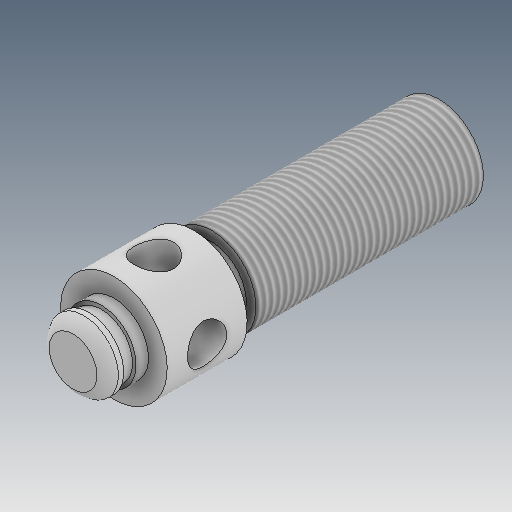
# Autodesk Inventor part: 螺杆
Saved by Autodesk Inventor 2020 (Build 240168000, 168)
## iProperties
Created: 2021-05-02
Part Number: 螺杆
Material: 常规
Document SubType Name: Modeling
Designer: Luorily
Density: 1 g/cm^3
Appearance: 默认
Author: Luorily
Autodesk Inventor part; units mm, degrees
ref_plane "YZ Plane" through (0, 0, 0) normal (1, 0, 0) x (0, 1, 0)
ref_plane "XZ Plane" through (0, 0, 0) normal (0, 1, 0) x (-1, 0, 0)
ref_plane "XY Plane" through (0, 0, 0) normal (0, 0, 1) x (1, 0, 0)
sketch "草图1" plane through (0, 0, 0) normal (1, 0, 0) x (0, 1, 0)
  line L0 (19.5, -23) -> (30, -23)
  line L1 (30, -23) -> (30, -68)
  line L2 (30, -68) -> (19.5, -68)
  line L3 (19.5, -68) -> (19.5, -78)
  line L4 (19.5, -78) -> (25, -78)
  line L5 (25, -78) -> (25, -206)
  line L6 (25, -206) -> (0, -206)
  line L7 (0, -206) -> (0, 0)
  line L8 (17.5, -16) -> (17.5, -9)
  line L9 (17.5, -9) -> (19.5, -9)
  line L10 (17.5, -16) -> (19.5, -16)
  line L11 (19.5, -16) -> (19.5, -23)
  line L12 (19.5, -23) -> (19.5, -6)
  line L13 (0, 0) -> (13.5, 0)
  arc A0 (19.5, -6) -> (13.5, 0) centre (8.1859, -11.3141) ccw
  dimension "d2" = 10.5
  dimension "d3" = 45
  dimension "d4" = 10.5
  dimension "d5" = 10
  dimension "d6" = 5.5
  dimension "d7" = 128
  dimension "d10" = 7
  dimension "d11" = 17
  dimension "d14" = 13.5
  dimension "d15" = 25
  constraints: 28 end point, 7 perpendicular, 2 parallel, 2 point on circle, 1 centre point, 1 horizontal
  measures "d2" distance of L0.start L0.end
  measures "d3" distance of L0.end L1.end
  measures "d4" distance of L1.end L2.end
  measures "d5" distance of L2.end L3.end
  measures "d6" distance of L3.end L4.end
  measures "d7" distance of L4.end L5.end
  measures "d10" distance of L8.start L8.end
  measures "d11" distance of L12.end L0.start
  measures "d14" distance of L7.end L13.end
  measures "d15" distance of L5.end L6.end
revolve "旋转1" add sketch "草图1" angle 360 about axis through (0, 0, -206) along (0, 0, 1) contours L0 L1 L2 L3 L4 L5 L6 L7 L13 A0 L12 L9 L8 L10 L11
sketch "草图2" plane through (0, 0, 0) normal (0, 1, 0) x (-1, 0, 0)
  line L0 (-19.5, -68) -> (19.5, -68) projected
  line L1 (0, -68) -> (0, -45.5)
  circle A0 centre (0, -45.5) radius 11
  point P0 (0, 0)
  dimension "d17" = 22.5
  dimension "d18" = 22
  constraints: 2 end point, 1 centre point, 1 coincident, 1 midpoint, 1 vertical
  measures "d17" distance of L1.start L1.end
  measures "d18" diameter of A0
extrude "拉伸1" cut sketch "草图2" along normal blind 100 and the other way blind 100
thread "螺纹1" size "M50x4" class "6g" standard "ANSI Metric M Profile" full length
sketch "草图3" plane through (0, 0, 0) normal (1, 0, 0) x (0, 1, 0)
  line L0 (-19.5, -68) -> (19.5, -68) projected
  line L1 (0, -68) -> (0, -45.5)
  circle A0 centre (0, -45.5) radius 11
  line L2 (-30, -34.5) -> (30, -34.5) projected
  point P0 (0, 0)
  dimension "d25" = 22.5
  dimension "d26" = 22
  constraints: 2 end point, 1 centre point, 1 coincident, 1 midpoint, 1 tangent, 1 vertical
  measures "d25" distance of L1.start L1.end
  measures "d26" diameter of A0
extrude "拉伸2" cut sketch "草图3" along normal blind 100 and the other way blind 50
